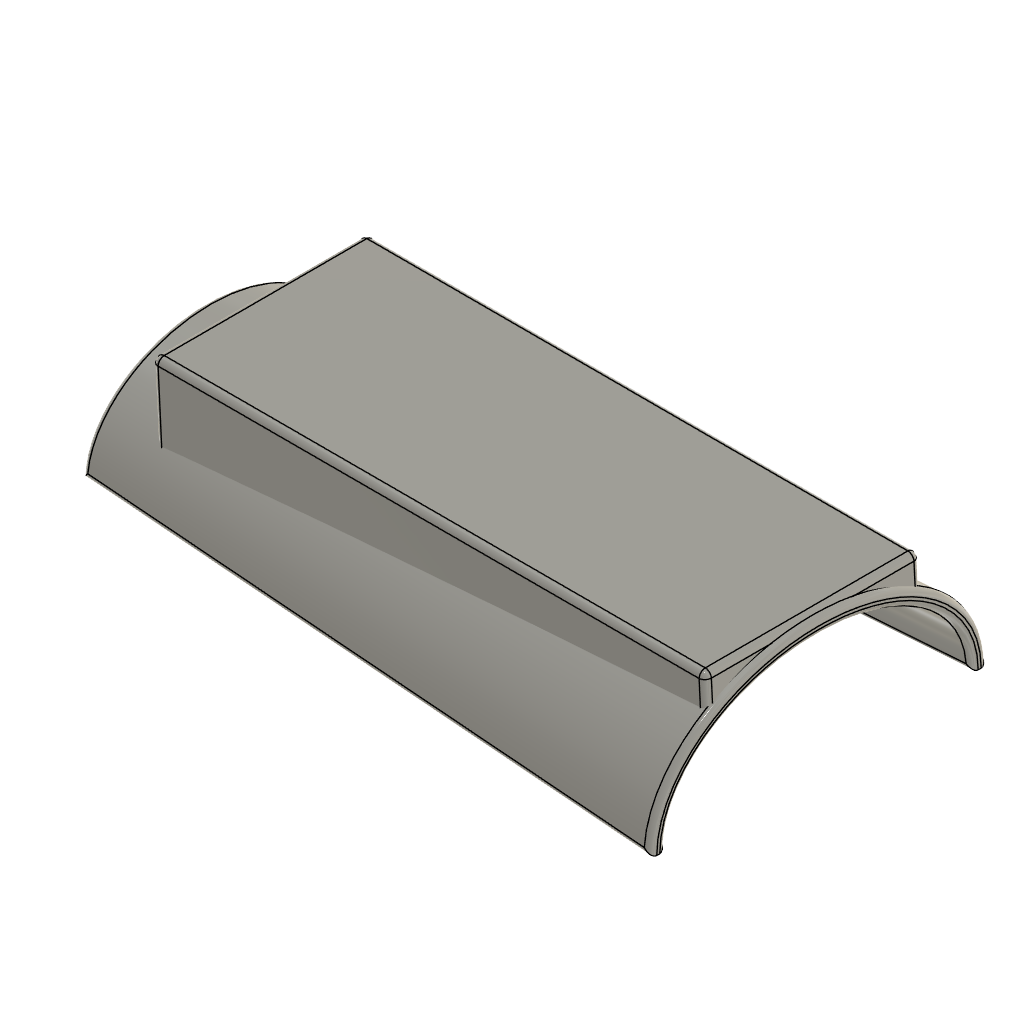
Soporte_Antebrazo (Autodesk Fusion 360 archive; units mm, degrees)
design "Soporte_Antebrazo"
part number: 2026-10-04-22-20-11-854
Autodesk Fusion 360 part; units mm, degrees
note: some values were not read from the file. Chosen so that the rebuilt part matches the saved one: which bodies a step acts on; which face or edge a step refers to.
sketch "Boceto1" plane through (0, 0, 0) normal (1, 0, 0) x (0, 1, 0)
  ellipse E0 centre (0, 0) end of major axis (-55, 0) minor radius 40.5
  line L0 (55, 0) -> (-55, 0) construction
  line L1 (0, 40.5) -> (0, -40.5) construction
  ellipse E1 centre (0, 0) end of major axis (-50, 0) minor radius 35.5
  line L2 (50, 0) -> (-50, 0) construction
  line L3 (0, 35.5) -> (0, -35.5) construction
  line L4 (55, 0) -> (-55, 0)
  dimension "d1" = 55
  dimension "d2" = 81
  dimension "d7" = 100
  dimension "d9" = 5
  dimension "d10" = 5
  dimension "d11" = 5
  constraint coincident E0 L0.start
  constraint coincident E0 L0.end
  constraint coincident E0 L1.start
  constraint coincident E0 L1.end
  constraint coincident E0.centre E1.centre
  constraint horizontal L0
  constraint coincident E1 L2.start
  constraint coincident E1 L2.end
  constraint coincident E1 L3.start
  constraint coincident E1 L3.end
  constraint concentric E0 E1
  constraint perpendicular L1 L2
  constraint coincident L0.start L4.start
  constraint coincident L0.end L4.end
  measures "d1" distance of E0
  measures "d7" distance of E1
  measures "d9" distance of L0.end L2.end
  measures "d10" distance of L1.start L3.start
  measures "d11" distance of L1.end L3.end
ref_plane "PlanoDeObra1" through (-200, 0, 0) normal (1, 0, 0) x (0, 1, 0)
sketch "Boceto2" plane through (-200, 0, 0) normal (1, 0, 0) x (0, 1, 0)
  ellipse E0 centre (0, 0) end of major axis (-40, 0) minor radius 30
  line L0 (40, 0) -> (-40, 0) construction
  line L1 (0, 30) -> (0, -30) construction
  ellipse E1 centre (0, 0) end of major axis (-35, 0) minor radius 25
  line L2 (35, 0) -> (-35, 0) construction
  line L3 (0, 25) -> (0, -25) construction
  line L4 (40, 0) -> (-40, 0)
  dimension "d5" = 40
  dimension "d6" = 30
  dimension "d12" = 70
  dimension "d13" = 5
  dimension "d14" = 5
  constraint coincident E0 L0.start
  constraint coincident E0 L0.end
  constraint coincident E0 L1.start
  constraint coincident E0 L1.end
  constraint coincident E0.centre E1.centre
  constraint horizontal L0
  constraint coincident E1 L2.start
  constraint coincident E1 L2.end
  constraint coincident E1 L3.start
  constraint coincident E1 L3.end
  constraint perpendicular L1 L2
  constraint coincident L0.start L4.start
  constraint coincident L0.end L4.end
  measures "d5" distance of E0
  measures "d12" distance of E1
  measures "d13" distance of L1.start L3.start
  measures "d14" distance of L1.end L3.end
loft "Solevación1" add profiles "Boceto2", "Boceto1" section 1 contours E0 E1 L4 picked at (4.7532, 28.0526) section 2 contours E0 E1 L4 picked at (-5.2315, 38.5622) makes body 1
fillet "Empalme1" radius 2 1 edges at (0, 0, 40.5) on bodies 1
fillet "Empalme1" radius 2 7 edges at (0, 0, 35.5) (-200, 0, 30) (-200, 0, 25) (-100, -47.5, 0) (-100, -42.5, 0) (-100, 42.5, 0) (-100, 47.5, 0) on bodies 1
ref_plane "PlanoDeObra2" through (0, 0, 40.5) normal (-0.052428, 0, 0.998625) x (0, -1, 0)
sketch "Boceto4" plane through (-2.1204, 0, 40.3887) normal (-0.052428, 0, 0.998625) x (0, -1, 0)
  line L0 (-35, 0) -> (35, 0)
  line L1 (35, 0) -> (35, -180)
  line L2 (35, -180) -> (-35, -180)
  line L3 (-35, -180) -> (-35, 0)
  point P0 (0, -180)
  point P1 (0, -198.1521)
  dimension "d22" = 180
  dimension "d23" = 70
  constraint horizontal L0
  constraint vertical L1
  constraint horizontal L2
  constraint vertical L3
  constraint midpoint L2 P0
  constraint midpoint L0 origin
  constraint collinear P0 origin P1
  measures "d22" distance of L0.start L2.end
  measures "d23" distance of L0.start L0.end
extrude "Extruir1" add sketch "Boceto4" along normal blind 20 and the other way blind 20 separate body makes body 2
ref_plane "PlanoDeObra4" through (0, 0, 41) normal (0, 0, 1) x (1, 0, 0)
split "Dividir1" by plane through (0, 0, 41) normal (0, 0, 1) bodies 2 makes body 3 at (-63.0864, -11.6667, 57.2155)
delete_body "QuitarCuerpo1" bodies 3
split "Dividir2" by face at (-67.2284, 0.4655, 31.9688) of body 1 bodies 2 makes body 4 at (-92.8956, -11.6667, 15.5954)
delete_body "QuitarCuerpo3" bodies 4
fillet "Empalme3" radius 2 8 edges at (-182.4004, 0, 41) (-181.6123, -35, 25.9896) (-181.6123, 35, 25.9896) (-92.2764, 35, 41) (-2.1525, 0, 41) (-1.7392, 35, 33.1269) (-1.7392, -35, 33.1269) (-92.2764, -35, 41) on bodies 2
